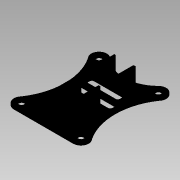
# Autodesk Inventor part: basebawahV2
Saved by Autodesk Inventor 2015 SP1 (Build 190203100, 203)
## iProperties
Created: 2015-01-14
Part Number: basebawahV2
Material: ABS Plastic
Document SubType Name: Modeling
Designer: Rafi Kurnia Putra
Density: 1.06 g/cm^3
Appearance: Default
Mass: 42.2508 g
Surface Area: 270.463 cm^2
Volume: 39.8593 cm^3
Author: Rafi Kurnia Putra
Autodesk Inventor part; units mm, degrees
ref_plane "YZ Plane" through (0, 0, 0) normal (1, 0, 0) x (0, 1, 0)
ref_plane "XZ Plane" through (0, 0, 0) normal (0, 1, 0) x (-1, 0, 0)
ref_plane "XY Plane" through (0, 0, 0) normal (0, 0, 1) x (1, 0, 0)
sketch "Sketch1" plane through (0, 0, 0) normal (0, 1, 0) x (-1, 0, 0)
  circle A0 centre (46.649975, 60.886623) radius 4.25
  circle A1 centre (25.374996, 42.175) radius 1.75
  circle A2 centre (28.624996, 37.55) radius 1.75
  circle A3 centre (46.649977, -60.886624) radius 4.25
  circle A4 centre (25.374996, -42.175) radius 1.75
  circle A5 centre (28.624996, -37.55) radius 1.75
  circle A6 centre (25.499998, -34.24) radius 1.75
  circle A7 centre (25.499998, 34.24) radius 1.75
  arc A8 (55.329713, 52.206889) -> (37.970237, 69.566356) centre (46.649975, 60.886623) ccw
  arc A9 (37.970237, -69.566356) -> (55.329713, -52.206889) centre (46.649975, -60.886623) ccw
  circle A10 centre (35.709129, 28.89871) radius 1.75
  circle A11 centre (38.62566, 37.55) radius 1.75
  circle A12 centre (28.87566, 53.55) radius 1.75
  line L0 (12.265914, 71.745147) -> (15.322444, 61.724857)
  arc A13 (22.16891, 58.629565) -> (37.970237, 69.566356) centre (0.002246, 107.538826) ccw
  arc A14 (15.322444, 61.724857) -> (22.16891, 58.629565) centre (20.104898, 63.183668) ccw
  circle A15 centre (-25.375, 42.175) radius 1.75
  circle A16 centre (-28.625, 37.55) radius 1.75
  circle A17 centre (-46.649979, 60.886623) radius 4.25
  circle A18 centre (-25.375, -42.175) radius 1.75
  circle A19 centre (-28.625, -37.55) radius 1.75
  circle A20 centre (-46.64998, -60.886624) radius 4.25
  circle A21 centre (-25.500002, -34.24) radius 1.75
  circle A22 centre (-25.500002, 34.24) radius 1.75
  arc A23 (-37.970241, 69.566356) -> (-55.329716, 52.206889) centre (-46.649979, 60.886623) ccw
  arc A24 (-55.329716, -52.206889) -> (-37.970241, -69.566356) centre (-46.649979, -60.886623) ccw
  circle A25 centre (-28.875664, 53.55) radius 1.75
  circle A26 centre (-38.625664, 37.55) radius 1.75
  circle A27 centre (-35.709132, 28.89871) radius 1.75
  line L1 (-12.265918, 71.745147) -> (-15.322448, 61.724857)
  arc A28 (-37.970241, 69.566356) -> (-22.168913, 58.629565) centre (-0.00225, 107.538826) ccw
  arc A29 (-22.168913, 58.629565) -> (-15.322448, 61.724857) centre (-20.104902, 63.183668) ccw
  circle A30 centre (-0.000002, 42.191238) radius 1.75
  arc A31 (37.970237, -69.566356) -> (-37.970241, -69.566356) centre (-0.000002, -107.52451) ccw
  line L2 (10.352933, 73.161623) -> (-10.352936, 73.161623)
  arc A32 (-55.329716, -52.206889) -> (-55.329716, 52.206889) centre (-134.113765, 0) ccw
  arc A33 (55.329713, 52.206889) -> (55.329713, -52.206889) centre (134.113761, 0) ccw
  arc A34 (12.265914, 71.745147) -> (10.352933, 73.161623) centre (10.352933, 71.161623) ccw
  arc A35 (-10.352936, 73.161623) -> (-12.265918, 71.745147) centre (-10.352936, 71.161623) ccw
  arc A36 (25.375, -21.859238) -> (21.875, -18.359238) centre (21.875, -21.859238) ccw
  arc A37 (21.875, -28.342705) -> (25.375, -24.842705) centre (21.875, -24.842705) ccw
  arc A38 (-25.374996, -24.842705) -> (-21.874996, -28.342705) centre (-21.874996, -24.842705) ccw
  arc A39 (-21.874996, -18.359238) -> (-25.374996, -21.859238) centre (-21.874996, -21.859238) ccw
  line L3 (-21.874996, -18.359238) -> (21.875, -18.359238)
  line L4 (21.875, -28.342705) -> (-21.874996, -28.342705)
  line L5 (-25.374996, -21.859238) -> (-25.374996, -24.842705)
  line L6 (25.375, -21.859238) -> (25.375, -24.842705)
  circle A40 centre (-0.000002, 61.161623) radius 1.25
  circle A41 centre (-0.000002, 66.161623) radius 1.25
  circle A42 centre (-0.000002, -42.191238) radius 1.75
  circle A43 centre (0, -48.013133) radius 1.75
  circle A44 centre (0, 48.013133) radius 1.75
  circle A45 centre (-34.62724, 13.898709) radius 1.75
  circle A46 centre (-34.62724, -13.89871) radius 1.75
  circle A47 centre (34.62724, 13.89871) radius 1.75
  circle A48 centre (34.62724, -13.89871) radius 1.75
  point P0 (57.609033, 54.428088)
  point P1 (16.895654, 56.567367)
  point P2 (-0.003539, -53.835028)
  point P3 (-57.609037, 54.428088)
  point P4 (-16.895657, 56.567367)
  point P5 (0.003535, -53.835028)
  point P6 (39.601934, 0)
  point P7 (-39.601937, 0)
  point P8 (25.25, -18.359238)
  point P9 (0.000004, -18.359238)
  point P10 (-25.249996, -18.359238)
  point P11 (46.649975, -73.161623)
  point P12 (-0.000002, -73.161623)
  point P13 (46.649975, 73.161623)
  point P14 (46.649975, -73.161623)
  point P15 (-40.629481, 13.89871)
  dimension "d105" = 3.5
  dimension "d106" = 3.5
  dimension "d198" = 16
  dimension "d199" = 8.65129
  dimension "d244" = 5
  dimension "d247" = 79.20387
  dimension "d248" = 2
  dimension "d249" = 3.5
  dimension "d250" = 2.5
  dimension "d251" = 2.5
  dimension "d252" = 146.32325
  dimension "d253" = 146.32325
  dimension "d258" = 6.00224
  dimension "d259" = 27.79742
  dimension "d260" = 69.25448
  dimension "d263" = 5.82189
  dimension "d264" = 5.8219
  dimension "d265" = 5.8219
  dimension "d266" = 46.98791
  dimension "d267" = 12.02274
  dimension "d271" = 46.98791
  dimension "d272" = 12.02274
  constraints: 49 centre point, 42 point on circle, 14 end point, 6 tangent, 3 coincident, 2 equal radius, 2 point on line, 1 horizontal, 1 parallel, 1 perpendicular, 2 other
  measures "d105" diameter of A6
  measures "d106" diameter of A7
  measures "d198" vertical distance of A12.centre A11.centre
  measures "d199" vertical distance of A10.centre A11.centre
  measures "d244" radius of A14
  measures "d247" distance of point (-39.602, 0) point (39.602, 0)
  measures "d248" radius of A34
  measures "d249" radius of A36
  measures "d250" diameter of A40
  measures "d251" diameter of A41
  measures "d252" distance from line of L2 point (0, -73.162)
  measures "d253" distance of point (46.65, -73.162) point (46.65, 73.162)
  measures "d258" distance of A45.centre point (-40.629, 13.899)
  measures "d259" distance of A46.centre A45.centre
  measures "d260" distance of A47.centre A45.centre
  measures "d263" distance of A43.centre point (-0.004, -53.835)
  measures "d264" distance of A42.centre A43.centre
  measures "d265" distance of A30.centre A44.centre
  measures "d266" vertical distance of A45.centre A17.centre
  measures "d267" horizontal distance of A45.centre A17.centre
  measures "d271" vertical distance of A46.centre A20.centre
  measures "d272" horizontal distance of A46.centre A20.centre
extrude "Extrusion14" add sketch "Sketch1" along normal mid plane 3
sketch "Sketch14" plane through (0, -1.5, 0) normal (0, -1, 0) x (1, 0, 0)
  line L0 (31.815, 0) -> (31.815, -5.951937)
  arc A0 (28.315, -9.451937) -> (31.815, -5.951937) centre (28.315, -5.951937) ccw
  arc A1 (28.315, -9.451937) -> (28.625, -9.438182) centre (28.315, -5.951937) ccw
  line L1 (28.315, -9.451937) -> (0.054398, -9.451937)
  line L2 (28.315, 9.451937) -> (0.054398, 9.451937)
  arc A2 (31.815, 5.951937) -> (28.315, 9.451937) centre (28.315, 5.951937) ccw
  line L3 (31.815, 0) -> (31.815, 5.951937)
  arc A3 (28.625, 9.438182) -> (28.315, 9.451937) centre (28.315, 5.951937) ccw
  line L4 (-28.314996, -9.451937) -> (-0.054394, -9.451937)
  line L5 (-31.814996, 0) -> (-31.814996, -5.951937)
  arc A4 (-31.814996, -5.951937) -> (-28.314996, -9.451937) centre (-28.314996, -5.951937) ccw
  arc A5 (-28.624996, -9.438182) -> (-28.314996, -9.451937) centre (-28.314996, -5.951937) ccw
  line L6 (-28.314998, 9.438182) -> (-0.054396, 9.445009)
  arc A6 (-28.314998, 9.438182) -> (-28.625866, 9.424351) centre (-28.315023, 5.938182) ccw
  arc A7 (-28.314998, 9.438182) -> (-31.814996, 5.951937) centre (-28.315023, 5.938182) ccw
  line L7 (-31.814996, 0) -> (-31.814996, 5.951937)
  line L8 (-28.314998, 9.438182) -> (28.625, 9.438182)
  line L9 (28.625, -9.438182) -> (-28.624996, -9.438182)
  line L10 (-31.814996, 5.951937) -> (-31.814996, -5.951937)
  line L11 (31.815, 5.951937) -> (31.815, -5.951937)
  point P0 (0, 0)
  point P1 (0.000002, 0)
  dimension "d268" = 63.63
  constraints: 24 end point, 20 point on circle, 8 centre point, 2 collinear, 2 parallel
  measures "d268" distance of L5.start L0.start
extrude "Extrusion15" cut sketch "Sketch14" against normal blind 3
sketch "Sketch15" plane through (0, 1.5, 0) normal (0, 1, 0) x (1, 0, 0)
  arc A0 (-46.649975, -73.161623) -> (-37.970237, -69.566356) centre (-46.649975, -60.886623) ccw
  arc A1 (-22.168909, -58.629564) -> (-37.970237, -69.566356) centre (-0.002246, -107.538826) ccw
  arc A2 (-15.322444, -61.724856) -> (-22.168909, -58.629564) centre (-20.104898, -63.183668) ccw
  line L0 (-15.322444, -61.724856) -> (-12.265914, -71.745147)
  arc A3 (-12.265914, -71.745147) -> (-10.352932, -73.161623) centre (-10.352932, -71.161623) ccw
  arc A4 (10.352937, -73.161623) -> (12.265918, -71.745147) centre (10.352937, -71.161623) ccw
  line L1 (12.265918, -71.745147) -> (15.322448, -61.724856)
  arc A5 (22.168914, -58.629564) -> (15.322448, -61.724856) centre (20.104902, -63.183668) ccw
  arc A6 (37.970241, -69.566356) -> (22.168914, -58.629564) centre (0.00225, -107.538826) ccw
  arc A7 (37.970241, -69.566356) -> (46.649979, -73.161623) centre (46.649979, -60.886623) ccw
  arc A8 (-46.649975, -73.161623) -> (-37.970237, -69.566356) centre (-46.649975, -60.886623) ccw
  line L2 (-46.649975, -73.161623) -> (-10.352932, -73.161623)
  line L3 (10.352937, -73.161623) -> (46.649979, -73.161623)
  line L4 (31.815, -5.951937) -> (31.815, 3.5)
  arc A9 (28.625, -9.438182) -> (31.815, -5.951937) centre (28.315, -5.951937) ccw
  line L5 (-28.314998, -9.438182) -> (28.625, -9.438182)
  arc A10 (-31.814996, -5.951937) -> (-28.314998, -9.438182) centre (-28.315023, -5.938182) ccw
  line L6 (-31.814996, 3.5) -> (-31.814996, -5.951937)
  line L7 (28.315, 0) -> (-28.314996, 0)
  arc A11 (28.315, 0) -> (31.815, 3.5) centre (28.315, 3.5) ccw
  arc A12 (-31.814996, 3.5) -> (-28.314996, 0) centre (-28.314996, 3.5) ccw
  dimension "d278" = 3.5
  dimension "d279" = 3.5
  constraints: 26 point on circle, 21 centre point, 16 end point, 4 tangent, 2 horizontal
  measures "d278" radius of A11
  measures "d279" radius of A12
extrude "Extrusion16" add sketch "Sketch15" against normal blind 3 contours A0 A1 A2 L0 A3 L2 | A4 L1 A5 A6 A7 L3
extrude "Extrusion17" add sketch "Sketch15" against normal blind 3 contours A9 L5 A10 L6 A12 L7 A11 L4
sketch "Sketch18" plane through (0, -1.5, 0) normal (0, -1, 0) x (1, 0, 0)
  arc A0 (23.835283, 3.818207) -> (25.559006, 5.541935) centre (22.377186, 7.000023) ccw
  line L0 (25.877174, 15.648734) -> (25.877186, 7.000028)
  line L1 (22.377191, 3.500023) -> (-22.377286, 3.499959)
  circle A1 centre (20.877184, 8.500021) radius 1.75
  circle A2 centre (-20.877184, 8.500021) radius 1.75
  point P0 (0, 0)
  dimension "d285" = 5
  dimension "d286" = 5
  constraints: 2 centre point
  measures "d285" distance from line of A1.centre L1
  measures "d286" distance from line of A1.centre L0
extrude "Extrusion18" cut sketch "Sketch18" against normal up to next
sketch "Sketch19" plane through (0, -1.5, 0) normal (0, -1, 0) x (1, 0, 0)
  circle A0 centre (-30, 64.661761) radius 1.75
  line L0 (0, 0) -> (0, 78.748235)
  line L1 (-36.745399, 69.661752) -> (36.745116, 69.661857)
  circle A1 centre (-9, 28.499978) radius 1.75
  line L2 (22.377191, 3.500023) -> (-22.377286, 3.499959)
  circle A2 centre (30, 64.661761) radius 1.75
  circle A3 centre (9, 28.499978) radius 1.75
  dimension "d289" = 3.5
  dimension "d300" = 30
  dimension "d301" = 5
  dimension "d302" = 3.5
  dimension "d303" = 25
  dimension "d304" = 9
  constraints: 6 end point, 4 centre point, 2 symmetric about line, 1 vertical, 8 other
  measures "d289" diameter of A0
  measures "d300" distance from line of A0.centre L0
  measures "d301" distance from line of A0.centre L1
  measures "d302" diameter of A1
  measures "d303" distance from line of A1.centre L2
  measures "d304" distance from line of L0 A1.centre
sketch "Sketch20" plane through (0, -1.5, 0) normal (0, -1, 0) x (1, 0, 0)
  circle A0 centre (-35.709129, 28.89871) radius 1.75
  circle A1 centre (-20.877184, 8.500021) radius 1.75
  circle A2 centre (20.877184, 8.500021) radius 1.75
  circle A3 centre (35.709132, 28.89871) radius 1.75
  circle A4 centre (-38.62566, 37.55) radius 1.75
  circle A5 centre (38.625664, 37.55) radius 1.75
  circle A6 centre (-28.87566, 53.55) radius 1.75
  circle A7 centre (28.875664, 53.55) radius 1.75
  point P0 (0, 0)
extrude "Extrusion19" add sketch "Sketch20" against normal blind 3
extrude "Extrusion20" cut sketch "Sketch19" against normal through all
sketch "Sketch21" plane through (0, 1.5, 0) normal (0, 1, 0) x (1, 0, 0)
  line L0 (13.5, -50.389389) -> (13.5, 54.708966)
  line L1 (-13.5, 54.034789) -> (-13.5, -50.389389)
  line L2 (16.5, -50.389389) -> (16.5, 55.149918)
  line L3 (-16.5, 55.165725) -> (-16.5, -50.389389)
  arc A0 (-16.5, 55.165725) -> (-13.5, 54.034789) centre (6.619106, 111.948621) ccw
  arc A1 (13.5, 54.708966) -> (16.5, 55.149918) centre (6.619106, 111.948621) ccw
  line L4 (13.5, -50.389389) -> (16.5, -50.389389)
  line L5 (-16.5, -50.389389) -> (-13.5, -50.389389)
  point P0 (0, 0)
  dimension "d309" = 16.5
  dimension "d310" = 13.5
  dimension "d311" = 13.5
  dimension "d312" = 16.5
  constraints: 12 end point, 4 point on circle, 4 vertical, 2 centre point, 1 horizontal
  measures "d309" distance from line of point (0, 0) L2
  measures "d310" distance from line of point (0, 0) L0
  measures "d311" distance from line of point (0, 0) L1
  measures "d312" distance from line of L3 point (0, 0)
extrude "Extrusion23" add sketch "Sketch21" along normal blind 23.5
sketch "Sketch23" plane through (0, 1.5, 0) normal (0, -1, 0) x (1, 0, 0)
  line L0 (13.5, 0) -> (16.5, 0)
  line L1 (13.5, 0) -> (13.5, -9.438182)
  line L2 (13.5, -9.438182) -> (16.5, -9.438182)
  line L3 (16.5, -9.438182) -> (16.5, 0)
  line L4 (13.5, -28.342705) -> (16.5, -28.342705)
  line L5 (16.5, -28.342705) -> (16.5, -18.359238)
  line L6 (16.5, -18.359238) -> (13.5, -18.359238)
  line L7 (13.5, -18.359238) -> (13.5, -28.342705)
  line L8 (-16.5, 0) -> (-13.5, 0)
  line L9 (-16.5, -9.438182) -> (-16.5, 0)
  line L10 (-16.5, -9.438182) -> (-13.5, -9.438182)
  line L11 (-13.5, 0) -> (-13.5, -9.438182)
  line L12 (-16.5, -28.342705) -> (-13.5, -28.342705)
  line L13 (-13.5, -18.359238) -> (-13.5, -28.342705)
  line L14 (-13.5, -18.359238) -> (-16.5, -18.359238)
  line L15 (-16.5, -28.342705) -> (-16.5, -18.359238)
  point P0 (0, 0)
extrude "Extrusion24" cut sketch "Sketch23" against normal through all
sketch "Sketch24" plane through (0, 25, 0) normal (0, 1, 0) x (1, 0, 0)
  line L0 (-16.5, 9.438182) -> (-13.5, 9.438182)
  line L1 (-13.5, 9.438182) -> (-13.5, 18.359238)
  line L2 (-13.5, 18.359238) -> (-16.5, 18.359238)
  line L3 (-16.5, 18.359238) -> (-16.5, 9.438182)
  line L4 (16.5, 18.359238) -> (13.5, 18.359238)
  line L5 (13.5, 18.359238) -> (13.5, 9.438182)
  line L6 (13.5, 9.438182) -> (16.5, 9.438182)
  line L7 (16.5, 9.438182) -> (16.5, 18.359238)
  point P0 (0, 0)
extrude "Extrusion25" cut sketch "Sketch24" against normal blind 23.5
body "Solid10"
